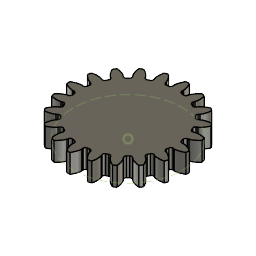
tyre (Autodesk Fusion 360 archive; units mm, degrees)
design "gear"
description: Spur Gear; Module: 2.000000; Num Teeth: 20; Pressure Angle: 20.000000; Backlash: 0.20 mm
Autodesk Fusion 360 part; units mm, degrees
sketch "Sketch1" plane through (0, 0, 0) normal (0, 0, 1) x (1, 0, 0) in component "Spur Gear (20 teeth)"
  circle A0 centre (0, 0) radius 17.5492
extrude "Extrude1" add sketch "Sketch1" along normal blind 7 in component "Spur Gear (20 teeth)"
sketch "Sketch2" plane through (0, 0, 0) normal (0, 0, 1) x (1, 0, 0) in component "Spur Gear (20 teeth)"
  spline S0 degree 5 poles (18.7162, -1.7068) (18.7256, -1.7077) (18.7444, -1.7091) (18.7726, -1.7106) (18.8102, -1.7111) (18.8573, -1.7097) (18.9045, -1.707) (18.9518, -1.7034) (18.999, -1.6994) (19.0463, -1.695) (19.0936, -1.6902) (19.1409, -1.6851) (19.1883, -1.6793) (19.2356, -1.6729) (19.2829, -1.6658) (19.3303, -1.658) (19.3776, -1.6497) (19.425, -1.641) (19.4723, -1.6318) (19.5197, -1.6223) (19.567, -1.6124) (19.6143, -1.6021) (19.6616, -1.5914) (19.7089, -1.5802) (19.7562, -1.5687) (19.8035, -1.5567) (19.8507, -1.5444) (19.898, -1.5316) (19.9452, -1.5186) (19.9924, -1.5051) (20.0396, -1.4914) (20.0867, -1.4773) (20.1339, -1.4628) (20.181, -1.448) (20.2281, -1.4329) (20.2752, -1.4174) (20.3222, -1.4016) (20.3692, -1.3854) (20.4162, -1.369) (20.4631, -1.3523) (20.5101, -1.3352) (20.557, -1.3178) (20.6038, -1.3001) (20.6506, -1.2822) (20.6974, -1.2639) (20.7442, -1.2453) (20.7909, -1.2264) (20.8376, -1.2073) (20.8843, -1.1878) (20.9309, -1.1681) (20.9774, -1.1481) (21.024, -1.1278) (21.0705, -1.1072) (21.1169, -1.0863) (21.1633, -1.0652) (21.2097, -1.0438) (21.256, -1.0221) (21.3023, -1.0002) (21.3485, -0.978) (21.3947, -0.9555) (21.4409, -0.9328) (21.487, -0.9098) (21.533, -0.8865) (21.579, -0.863) (21.625, -0.8392) (21.6709, -0.8151) (21.7167, -0.7909) (21.7625, -0.7663) (21.8083, -0.7415) (21.8539, -0.7165) (21.8996, -0.6912) (21.9361, -0.6707) (21.9634, -0.6553) (21.9816, -0.645) (21.9907, -0.6398) knots 0 0 0 0 0 0 0.01428571 0.02857143 0.04285714 0.05714286 0.07142857 0.08571429 0.1 0.11428571 0.12857143 0.14285714 0.15714286 0.17142857 0.18571429 0.2 0.21428571 0.22857143 0.24285714 0.25714286 0.27142857 0.28571429 0.3 0.31428571 0.32857143 0.34285714 0.35714286 0.37142857 0.38571429 0.4 0.41428571 0.42857143 0.44285714 0.45714286 0.47142857 0.48571429 0.5 0.51428571 0.52857143 0.54285714 0.55714286 0.57142857 0.58571429 0.6 0.61428571 0.62857143 0.64285714 0.65714286 0.67142857 0.68571429 0.7 0.71428571 0.72857143 0.74285714 0.75714286 0.77142857 0.78571429 0.8 0.81428571 0.82857143 0.84285714 0.85714286 0.87142857 0.88571429 0.9 0.91428571 0.92857143 0.94285714 0.95714286 0.97142857 0.98571429 1 1 1 1 1 1
  spline S1 degree 5 poles (18.7162, 1.7068) (18.7256, 1.7077) (18.7444, 1.7091) (18.7726, 1.7106) (18.8102, 1.7111) (18.8573, 1.7097) (18.9045, 1.707) (18.9518, 1.7034) (18.999, 1.6994) (19.0463, 1.695) (19.0936, 1.6902) (19.1409, 1.6851) (19.1883, 1.6793) (19.2356, 1.6729) (19.2829, 1.6658) (19.3303, 1.658) (19.3776, 1.6497) (19.425, 1.641) (19.4723, 1.6318) (19.5197, 1.6223) (19.567, 1.6124) (19.6143, 1.6021) (19.6616, 1.5914) (19.7089, 1.5802) (19.7562, 1.5687) (19.8035, 1.5567) (19.8507, 1.5444) (19.898, 1.5316) (19.9452, 1.5186) (19.9924, 1.5051) (20.0396, 1.4914) (20.0867, 1.4773) (20.1339, 1.4628) (20.181, 1.448) (20.2281, 1.4329) (20.2752, 1.4174) (20.3222, 1.4016) (20.3692, 1.3854) (20.4162, 1.369) (20.4631, 1.3523) (20.5101, 1.3352) (20.557, 1.3178) (20.6038, 1.3001) (20.6506, 1.2822) (20.6974, 1.2639) (20.7442, 1.2453) (20.7909, 1.2264) (20.8376, 1.2073) (20.8843, 1.1878) (20.9309, 1.1681) (20.9774, 1.1481) (21.024, 1.1278) (21.0705, 1.1072) (21.1169, 1.0863) (21.1633, 1.0652) (21.2097, 1.0438) (21.256, 1.0221) (21.3023, 1.0002) (21.3485, 0.978) (21.3947, 0.9555) (21.4409, 0.9328) (21.487, 0.9098) (21.533, 0.8865) (21.579, 0.863) (21.625, 0.8392) (21.6709, 0.8151) (21.7167, 0.7909) (21.7625, 0.7663) (21.8083, 0.7415) (21.8539, 0.7165) (21.8996, 0.6912) (21.9361, 0.6707) (21.9634, 0.6553) (21.9816, 0.645) (21.9907, 0.6398) knots 0 0 0 0 0 0 0.01428571 0.02857143 0.04285714 0.05714286 0.07142857 0.08571429 0.1 0.11428571 0.12857143 0.14285714 0.15714286 0.17142857 0.18571429 0.2 0.21428571 0.22857143 0.24285714 0.25714286 0.27142857 0.28571429 0.3 0.31428571 0.32857143 0.34285714 0.35714286 0.37142857 0.38571429 0.4 0.41428571 0.42857143 0.44285714 0.45714286 0.47142857 0.48571429 0.5 0.51428571 0.52857143 0.54285714 0.55714286 0.57142857 0.58571429 0.6 0.61428571 0.62857143 0.64285714 0.65714286 0.67142857 0.68571429 0.7 0.71428571 0.72857143 0.74285714 0.75714286 0.77142857 0.78571429 0.8 0.81428571 0.82857143 0.84285714 0.85714286 0.87142857 0.88571429 0.9 0.91428571 0.92857143 0.94285714 0.95714286 0.97142857 0.98571429 1 1 1 1 1 1
  arc A0 (21.9907, -0.6398) -> (21.9907, 0.6398) centre (0, 0) ccw
  line L0 (17.4667, -1.5938) -> (18.7162, -1.7068)
  line L1 (17.4667, 1.5938) -> (18.7162, 1.7068)
  line L2 (17.4667, -1.5938) -> (17.4667, 1.5938)
  point P0 (18.9464, -1.7037)
  point P1 (19.1784, -1.6804)
  point P2 (19.4114, -1.6434)
  point P3 (19.6452, -1.595)
  point P4 (19.8796, -1.5365)
  point P5 (20.1144, -1.4687)
  point P6 (20.3494, -1.3922)
  point P7 (20.5845, -1.3074)
  point P8 (20.8195, -1.2147)
  point P9 (21.0545, -1.1142)
  point P10 (21.2892, -1.0064)
  point P11 (21.5235, -0.8912)
  point P12 (21.7574, -0.769)
  point P13 (18.9464, 1.7037)
  point P14 (19.1784, 1.6804)
  point P15 (19.4114, 1.6434)
  point P16 (19.6452, 1.595)
  point P17 (19.8796, 1.5365)
  point P18 (20.1144, 1.4687)
  point P19 (20.3494, 1.3922)
  point P20 (20.5845, 1.3074)
  point P21 (20.8195, 1.2147)
  point P22 (21.0545, 1.1142)
  point P23 (21.2892, 1.0064)
  point P24 (21.5235, 0.8912)
  point P25 (21.7574, 0.769)
extrude "Extrude2" add sketch "Sketch2" along normal blind 7 in component "Spur Gear (20 teeth)"
fillet "Fillet1" radius 0.75 2 edges at (17.4766, -1.5947, 3.5) (17.4766, 1.5947, 3.5) in component "Spur Gear (20 teeth)"
pattern_circular "C-Pattern1" count 20 over 360 about axis through (0, 0, 0) along (0, 0, 1) of "Extrude2", "Fillet1" in component "Spur Gear (20 teeth)"
sketch "Sketch3" plane through (0, 0, 0) normal (0, 0, 1) x (1, 0, 0) in component "Spur Gear (20 teeth)"
  circle A0 centre (0, 0) radius 20 construction
component "Spur Gear (20 teeth)" placed x (1, 0, 0) y (0, 1, 0) z (0, 0, 1) at (0, 0, 0)
